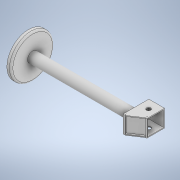
# Autodesk Inventor part: مهمه 4
Saved by Autodesk Inventor 2022 (Build 260153000, 153)
## iProperties
Created: 2021-07-15
Part Number: مهمه 4
Material: Generic
Document SubType Name: Modeling
Designer: Nay
Density: 1 g/cm^3
Appearance: Default
Author: Nay
Autodesk Inventor part; units mm, degrees
ref_plane "YZ Plane" through (0, 0, 0) normal (1, 0, 0) x (0, 1, 0)
ref_plane "XZ Plane" through (0, 0, 0) normal (0, 1, 0) x (-1, 0, 0)
ref_plane "XY Plane" through (0, 0, 0) normal (0, 0, 1) x (1, 0, 0)
sketch "Sketch1" plane through (0, 0, 0) normal (1, 0, 0) x (0, 1, 0)
  circle A0 centre (0, 0) radius 25
  dimension "d0" = 50
  constraints: 1 centre point, 1 coincident
  measures "d0" diameter of A0
extrude "Extrusion1" add sketch "Sketch1" along normal blind 5
fillet "Fillet1" radius 2 1 edges at (5, -25, 0)
sketch "Sketch2" plane through (5, 0, 0) normal (1, 0, 0) x (0, 0, -1)
  circle A0 centre (0, 0) radius 6
  dimension "d4" = 12
  constraints: 1 centre point, 1 coincident
  measures "d4" diameter of A0
extrude "Extrusion2" add sketch "Sketch2" along normal blind 120
sketch "Sketch3" plane through (125, 0, 0) normal (1, 0, 0) x (0, 0, -1)
  line L0 (15, 10) -> (-15, 10)
  line L1 (-15, 10) -> (-15, -10)
  line L2 (-15, -10) -> (15, -10)
  line L3 (15, -10) -> (15, 10)
  point P0 (0, 0)
  dimension "d7" = 20
  dimension "d8" = 30
  dimension "d9" = 15
  dimension "d10" = 10
  constraints: 8 end point, 2 parallel, 1 horizontal, 1 perpendicular
  measures "d7" distance of L2.end L0.start
  measures "d8" distance of L1.end L2.end
  measures "d9" distance from line of point (0, 0) L3
  measures "d10" distance from line of L0 point (0, 0)
extrude "Extrusion3" add sketch "Sketch3" along normal blind 20
sketch "Sketch4" plane through (145, 0, 0) normal (1, 0, 0) x (0, 0, -1)
  line L0 (-14, -9) -> (14, -9)
  line L1 (14, -9) -> (14, 9)
  line L2 (14, 9) -> (-14, 9)
  line L3 (-14, 9) -> (-14, -9)
  line L4 (-15, -10) -> (15, -10) projected
  line L5 (15, -10) -> (15, 10) projected
  point P0 (0, 0)
  dimension "d13" = 28
  dimension "d14" = 18
  dimension "d15" = 1
  dimension "d16" = 1
  constraints: 8 end point, 2 parallel, 1 horizontal, 1 perpendicular
  measures "d13" distance of L0.start L0.end
  measures "d14" distance of L2.end L0.start
  measures "d15" distance between parallel lines of L0 L4
  measures "d16" distance between parallel lines of L5 L1
extrude "Extrusion4" cut sketch "Sketch4" against normal blind 19
sketch "Sketch5" plane through (125, 10, 15) normal (0, 1, 0) x (1, 0, 0)
  line L0 (0, 0) -> (20, 0) projected
  line L1 (2.7176, 0) -> (1.4771, 2.1348)
  line L2 (1.4771, 2.1348) -> (16.6105, 12.2356)
  line L3 (16.6105, 12.2356) -> (18.2313, 9.8073)
  line L4 (18.2313, 9.8073) -> (18.2313, 30)
  line L5 (0, 30) -> (20, 30) projected
  line L6 (20, 30) -> (20, 0) projected
  line L7 (20, 30) -> (20, 0)
  line L8 (20, 0) -> (2.7176, 0)
  point P0 (-125, 15)
  constraints: 12 end point, 2 perpendicular, 2 point on line, 2 vertical
extrude "Extrusion5" cut sketch "Sketch5" against normal blind 30
sketch "Sketch6" plane through (141.6105, 9, 2.7644) normal (0.5551496, 0, 0.8317505) x (0.8317505, 0, -0.5551496)
  line L0 (-18.1947, 1) -> (0, 1) projected
  line L1 (0, -19) -> (-18.1947, -19) projected
  line L2 (0, 1) -> (-18.1947, 1)
  line L3 (-18.1947, 1) -> (-18.1947, -19)
  line L4 (-18.1947, -19) -> (0, -19)
  line L5 (0, -19) -> (0, 1)
  point P0 (-116.25, -9)
  constraints: 8 end point, 2 parallel, 1 horizontal, 1 perpendicular
extrude "Extrusion6" add sketch "Sketch6" along normal blind 0.5
sketch "Sketch7" plane through (125, -10, -15) normal (0, -1, 0) x (1, 0, 0)
  circle A0 centre (9.8115, 10.087) radius 2.5
  point P0 (-125, 15)
  dimension "d23" = 5
  constraints: 1 centre point
  measures "d23" diameter of A0
extrude "Extrusion7" cut sketch "Sketch7" against normal blind 25
sketch "Sketch8" plane through (143.2313, -10, 5.1927) normal (-0.8317505, 0, 0.5551496) x (0.5551496, 0, 0.8317505)
  line L0 (-16.7953, 0) -> (0, 0) projected
  line L1 (0, 20) -> (-16.7953, 20) projected
  line L2 (0, 0) -> (-2.3419, 0)
  line L3 (-2.3419, 0) -> (-2.3419, 20)
  line L4 (-2.3419, 20) -> (0, 20)
  line L5 (0, 20) -> (0, 0)
  point P0 (-83.8338, 10)
  point P1 (-2.3419, 0)
  constraints: 8 end point, 2 parallel, 1 horizontal, 1 perpendicular, 1 point on line
extrude "Extrusion8" add sketch "Sketch8" along normal blind 1
sketch "Sketch9" plane through (141.8881, 9, 3.1803) normal (0.5551496, 0, 0.8317505) x (0.8317505, 0, -0.5551496)
  line L0 (-18.1947, -19) -> (-18.3481, -19) projected
  line L1 (-18.1947, -18) -> (0, -18) projected
  line L2 (-18.1947, -19) -> (-0.9871, -19)
  line L3 (-0.9871, -19) -> (-0.9871, -18)
  line L4 (-0.9871, -18) -> (-18.1947, -18)
  line L5 (-18.1947, -18) -> (-18.1947, -19)
  point P0 (-116.25, -9)
  point P1 (-18.1947, -18)
  constraints: 8 end point, 2 parallel, 1 horizontal, 1 perpendicular, 1 point on line
extrude "Extrusion9" add sketch "Sketch9" along normal blind 2
sketch "Sketch10" plane through (141.8881, 9, 3.1803) normal (0.5551496, 0, 0.8317505) x (0.8317505, 0, -0.5551496)
  line L0 (-18.1947, 1) -> (-18.1947, -18) projected
  line L1 (1.107, 0) -> (-3.893, 0) projected
  line L2 (-18.1947, 1) -> (-0.936, 1)
  line L3 (-0.936, 1) -> (-0.936, 0)
  line L4 (-0.936, 0) -> (-18.1947, 0)
  line L5 (-18.1947, 0) -> (-18.1947, 1)
  point P0 (-116.25, -9)
  point P1 (-3.893, 0)
  constraints: 8 end point, 2 parallel, 1 horizontal, 1 perpendicular, 1 point on line
extrude "Extrusion10" add sketch "Sketch10" along normal blind 2
body "Solid1"
